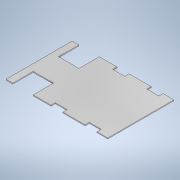
# Autodesk Inventor part: BottomSheet
Saved by Autodesk Inventor 2022 (Build 260153000, 153)
## iProperties
Created: 2022-01-11
Part Number: BottomSheet
Material: Generic
Document SubType Name: Modeling
Designer: Daniel Marquez
Density: 1 g/cm^3
Appearance: Aluminum - Polished
Author: Daniel Marquez
Autodesk Inventor part; units mm, degrees
ref_plane "YZ Plane" through (0, 0, 0) normal (1, 0, 0) x (0, 1, 0)
ref_plane "XZ Plane" through (0, 0, 0) normal (0, 1, 0) x (-1, 0, 0)
ref_plane "XY Plane" through (0, 0, 0) normal (0, 0, 1) x (1, 0, 0)
sketch "Sketch1" plane through (0, 0, 0) normal (0, 1, 0) x (-1, 0, 0)
  line L0 (711.2, -95.25) -> (711.2, -247.65)
  line L1 (711.2, -95.25) -> (558.8, -95.25)
  line L2 (170.18, -215.9) -> (170.18, -247.65)
  line L3 (170.18, -247.65) -> (336.55, -247.65)
  line L4 (336.55, -247.65) -> (336.55, -215.9)
  line L5 (711.2, -247.65) -> (762, -247.65)
  line L6 (170.18, -215.9) -> (81.28, -215.9)
  line L7 (81.28, -215.9) -> (81.28, -247.65)
  line L8 (81.28, -247.65) -> (0, -247.65)
  line L9 (762, -247.65) -> (762, 0)
  line L10 (0, 0) -> (0, -247.65)
  line L11 (336.55, -215.9) -> (425.45, -215.9)
  line L12 (558.8, -95.25) -> (558.8, -247.65)
  line L13 (558.8, -247.65) -> (425.45, -247.65)
  line L14 (425.45, -247.65) -> (425.45, -215.9)
  line L15 (848.7626, 0) -> (-141.8374, 0) construction
  line L16 (711.2, 95.25) -> (711.2, 247.65)
  line L17 (711.2, 95.25) -> (558.8, 95.25)
  line L18 (170.18, 215.9) -> (170.18, 247.65)
  line L19 (170.18, 247.65) -> (336.55, 247.65)
  line L20 (336.55, 247.65) -> (336.55, 215.9)
  line L21 (711.2, 247.65) -> (762, 247.65)
  line L22 (170.18, 215.9) -> (81.28, 215.9)
  line L23 (81.28, 215.9) -> (81.28, 247.65)
  line L24 (81.28, 247.65) -> (0, 247.65)
  line L25 (762, 247.65) -> (762, 0)
  line L26 (0, 0) -> (0, 247.65)
  line L27 (336.55, 215.9) -> (425.45, 215.9)
  line L28 (558.8, 95.25) -> (558.8, 247.65)
  line L29 (558.8, 247.65) -> (425.45, 247.65)
  line L30 (425.45, 247.65) -> (425.45, 215.9)
  dimension "d129" = 762
  dimension "d130" = 711.2
  dimension "d134" = 170.18
  dimension "d135" = 81.28
  dimension "d139" = 31.75
  dimension "d141" = 336.55
  dimension "d143" = 0
  dimension "d144" = 152.4
  dimension "d145" = 31.75
  dimension "d147" = 31.75
  dimension "d148" = 133.35
  dimension "d149" = 990.6
  constraints: 62 end point, 14 symmetric about line, 6 perpendicular, 5 horizontal, 2 vertical
  measures "d129" distance between parallel lines of L10 L9
  measures "d130" distance between parallel lines of L10 L0
  measures "d134" distance between parallel lines of L10 L2
  measures "d135" distance between parallel lines of L10 L7
  measures "d139" distance between parallel lines of L3 L6
  measures "d141" distance between parallel lines of L10 L4
  measures "d143" distance between parallel lines of L3 L8
  measures "d144" distance between parallel lines of L5 L1
  measures "d145" distance of L3.end L4.end
  measures "d147" distance between parallel lines of L13 L11
  measures "d148" distance between parallel lines of L12 L14
  measures "d149" distance of L15.start L15.end
extrude "Extrusion1" add sketch "Sketch1" along normal blind 6.35
body "Solid1"
